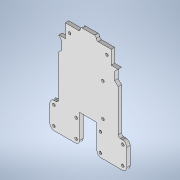
# Autodesk Inventor part: Основа робота
Saved by Autodesk Inventor 2020 (Build 240168000, 168)
## iProperties
Created: 2021-02-28
Part Number: Основа робота
Material: Типовые
Document SubType Name: Обычные детали
Designer: Антон
Density: 1 g/cm^3
Appearance: По умолчанию
Mass: 52.0111 g
Surface Area: 352.197 cm^2
Volume: 52.0111 cm^3
Sheet Metal Rule: По умолчанию
Author: Антон
Autodesk Inventor part; units mm, degrees
ref_plane "YZ Plane" through (0, 0, 0) normal (1, 0, 0) x (0, 1, 0)
ref_plane "XZ Plane" through (0, 0, 0) normal (0, 1, 0) x (-1, 0, 0)
ref_plane "XY Plane" through (0, 0, 0) normal (0, 0, 1) x (1, 0, 0)
sketch "Эскиз1" plane through (0, 0, 0) normal (0, 0, 1) x (1, 0, 0)
  line L0 (0, 0) -> (34.5, 0)
  line L1 (34.5, 0) -> (34.5, 114.55)
  line L2 (34.5, 114.55) -> (0, 114.55)
  line L3 (0, 114.55) -> (0, 0)
  line L4 (0, 0) -> (-9.9, 0)
  line L5 (-9.9, 0) -> (-9.9, 30.3)
  line L6 (-9.9, 30.3) -> (0, 30.3)
  line L7 (0, 30.3) -> (0, 0)
  line L8 (-9.9, 0) -> (-5.35, 0)
  line L9 (-5.35, 0) -> (-5.35, 4.55)
  line L10 (-5.35, 4.55) -> (-5.35, 25.75)
  circle A0 centre (-5.35, 25.75) radius 1.6
  circle A1 centre (-5.35, 4.55) radius 1.6
  line L11 (34.5, 0) -> (24.5, 0)
  line L12 (24.5, 0) -> (24.5, 33)
  line L13 (24.5, 33) -> (34.5, 33)
  line L14 (34.5, 33) -> (34.5, 0)
  line L15 (24.5, 4.55) -> (20.5, 4.55)
  line L16 (24.5, 25.75) -> (20.5, 25.75)
  circle A2 centre (20.5, 25.75) radius 1.6
  circle A3 centre (20.5, 4.55) radius 1.6
  line L17 (34.5, 114.55) -> (34.5, 114.55)
  line L18 (34.5, 114.55) -> (18, 114.55)
  line L19 (20.5, 25.75) -> (20.5, 4.55)
  circle A4 centre (12.95, 106.55) radius 1.6
  line L20 (8, 114.55) -> (8, 98.55)
  line L21 (8, 98.55) -> (0, 98.55)
  line L22 (0, 98.55) -> (0, 129.6)
  line L23 (34.5, 114.55) -> (25.25, 114.55)
  line L24 (25.25, 114.55) -> (25.25, 119)
  line L25 (25.25, 119) -> (34.5, 119)
  line L26 (34.5, 119) -> (34.5, 114.55)
  line L27 (0, 98.55) -> (4, 94.55)
  line L28 (4, 94.55) -> (4, 85.125)
  line L29 (4, 85.125) -> (0, 81.125)
  point P0 (0, 30.3)
  point P1 (34.5, 33)
  point P2 (0, 182.1)
  point P3 (20.5, 15.15)
  point P4 (-5.35, 15.15)
  point P5 (0, 98.55)
  point P6 (8, 106.55)
  point P7 (0, 114.55)
  dimension "d0" = 34.5
  dimension "d1" = 114.55
  dimension "d191" = 9.9
  dimension "d192" = 30.3
  dimension "d207" = 4.55
  dimension "d208" = 4.55
  dimension "d209" = 21.2
  dimension "d210" = 10
  dimension "d211" = 33
  dimension "d215" = 4
  dimension "d290" = 3.2
  dimension "d387" = 21.2
  dimension "d418" = 4.55
  dimension "d421" = 3.2
  dimension "d427" = 8
  dimension "d428" = 16
  dimension "d433" = 4.95
  dimension "d448" = 9.25
  dimension "d450" = 4.45
  dimension "d453" = 45
  dimension "d454" = 4
  dimension "d455" = 17.425
  constraints: 60 end point, 10 parallel, 8 perpendicular, 8 point on line, 6 horizontal, 5 centre point, 4 coincident, 3 equal radius, 3 midpoint, 2 collinear, 2 horizontal alignment, 2 vertical
  measures "d0" distance of L2.end L1.end
  measures "d1" distance of L1.end L0.end
  measures "d191" distance of L5.end L6.end
  measures "d192" distance of L4.end L5.end
  measures "d207" distance of L4.end L8.end
  measures "d208" distance of L8.end L9.end
  measures "d209" distance of L9.end L10.end
  measures "d210" distance of L12.end L13.end
  measures "d211" distance of L11.end L12.end
  measures "d215" distance of L16.start L16.end
  measures "d290" diameter of A2
  measures "d387" distance of L19.end L19.start
  measures "d418" distance from line of L0 L15.end
  measures "d421" diameter of A4
  measures "d427" distance of L20.end L21.end
  measures "d428" distance of L20.start L20.end
  measures "d433" distance of A4.centre point (8, 106.55)
  measures "d448" distance of L24.end L25.end
  measures "d450" distance of L23.end L24.end
  measures "d453" angle of L3 L29
  measures "d454" distance between parallel lines of L3 L28
  measures "d455" distance of L21.end L29.end
extrude "Выдавливание1" add sketch "Эскиз1" along normal blind 4 contours L3 L29 L28 L27 L21 L20 L2 L1 L13 L12 L16 A2 L19 A3 L15 L0 | L4 L5 L6 L3 | L15 A3 L19 A2 L16 L12 | L2 L24 L25 L26
mirror "Зеркальное отражение1" about plane through (34.5, 33, 0) normal (1, 0, 0)
sketch "Эскиз32" plane through (0, 0, 4) normal (0, 0, 1) x (1, 0, 0)
  line L0 (24.5, 33) -> (34.5, 33) construction
  line L1 (34.5, 33) -> (34.5, 39.862) construction
  line L2 (34.5, 39.862) -> (51.4, 39.862) construction
  line L3 (51.4, 39.862) -> (51.4, 78.087) construction
  point P0 (0, 0)
  point P1 (44.5, 33)
  dimension "d434" = 6.862
  dimension "d435" = 16.9
  dimension "d451" = 38.225
  constraints: 7 end point, 2 vertical, 1 horizontal
  measures "d434" distance of L0.end L1.end
  measures "d435" distance of L1.end L2.end
  measures "d451" distance of L2.end L3.end
hole "Отверстие14" at (51.4, 39.862, 4) at (51.4, 78.087, 4) direction (0, 0, -1) diameter 3.2 end through all
fillet "Сопряжение13" radius 2.225 4 edges at (25.25, 114.55, 2) (25.25, 119, 2) (43.75, 114.55, 2) (43.75, 119, 2)
fillet "Сопряжение2" radius 5.05 6 edges at (-9.9, 30.3, 2) (-9.9, 0, 2) (24.5, 0, 2) (44.5, 0, 2) (78.9, 0, 2) (78.9, 30.3, 2)
sketch "Эскиз19" plane through (0, 0, 0) normal (0, 0, -1) x (-1, 0, 0)
  line L0 (-15.75, 108.1666) -> (-12.95, 109.7832)
  line L1 (-12.95, 109.7832) -> (-10.15, 108.1666)
  line L2 (-10.15, 108.1666) -> (-10.15, 104.9334)
  line L3 (-10.15, 104.9334) -> (-12.95, 103.3168)
  line L4 (-12.95, 103.3168) -> (-15.75, 104.9334)
  line L5 (-15.75, 104.9334) -> (-15.75, 108.1666)
  line L6 (0, 81.125) -> (0, 30.3) projected
  circle A0 centre (-12.95, 106.55) radius 1.6 projected
  point P0 (0, 139.6)
  point P1 (-78, 139.6)
  point P2 (-14, 129.6)
  point P3 (-64, 129.6)
  point P4 (0, 119.25)
  point P5 (0, 97.45)
  point P6 (0, 129.6)
  point P7 (-78, 129.6)
  point P8 (-8, 114.55)
  point P9 (-61, 114.55)
  dimension "d423" = 5.6
  constraints: 12 end point, 1 coincident, 1 parallel, 14 other
  measures "d423" distance between parallel lines of L2 L5
extrude "Выдавливание7" cut sketch "Эскиз19" against normal blind 2.6 contours L0 L1 L2 L3 L4 L5 | A0
fillet "Сопряжение12" radius 2.725 2 edges at (69, 30.3, 2) (0, 30.3, 2)
sketch "Эскиз25" plane through (0, 0, 0) normal (0, 0, -1) x (-1, 0, 0)
  circle A0 centre (-20.5, 25.75) radius 1.6 projected
  circle A1 centre (-20.5, 4.55) radius 1.6 projected
  circle A2 centre (5.35, 25.75) radius 1.6 projected
  circle A3 centre (5.35, 4.55) radius 1.6 projected
  circle A4 centre (-48.5, 25.75) radius 1.6 projected
  circle A5 centre (-48.5, 4.55) radius 1.6 projected
  circle A6 centre (-74.35, 4.55) radius 1.6 projected
  circle A7 centre (-74.35, 25.75) radius 1.6 projected
  circle A8 centre (-56.05, 106.55) radius 1.6 projected
  circle A9 centre (-56.05, 106.55) radius 1.6 projected
  circle A10 centre (-51.4, 39.862) radius 1.6 projected
  circle A11 centre (-51.4, 39.862) radius 1.6 projected
  circle A12 centre (-51.4, 78.087) radius 1.6 projected
  point P0 (0, 0)
  constraints: 11 coincident
pattern_sketch "Массив по эскизу1" of "Выдавливание7" from (12.95, 106.55, 0) copies at (20.5, 25.75, 0) at (20.5, 4.55, 0) at (-5.35, 25.75, 0) at (-5.35, 4.55, 0) at (48.5, 25.75, 0) at (48.5, 4.55, 0) at (74.35, 4.55, 0) at (74.35, 25.75, 0) at (56.05, 106.55, 0) at (51.4, 39.862, 0) at (51.4, 78.087, 0)
fillet "Сопряжение11" radius 0.2 1 edges at (0, 98.55, 2)
sketch "Эскиз31" plane through (0, 0, 0) normal (0, 0, -1) x (-1, 0, 0)
  line L0 (-69, 98.55) -> (0, 98.55) construction
  line L1 (0, 98.55) -> (0, 33) construction
  line L2 (0, 33) -> (-69, 33) construction
  line L3 (-69, 33) -> (-69, 98.55) construction
  line L4 (-61, 98.55) -> (-69, 98.55) projected
  line L5 (-69, 81.125) -> (-69, 30.3) projected
  line L6 (0, 81.125) -> (0, 30.3) projected
  line L7 (-24.5, 33) -> (-44.5, 33) projected
  point P0 (0, 0)
  point P1 (-69, 97.45)
  point P2 (-69, 32.99)
  point P3 (0, 97.45)
  point P4 (-34.5, 33)
  constraints: 3 collinear, 1 horizontal, 3 other
equation "\"Радиус_гибки\" = Толщина"
equation "\"Ширина_просечки\" = Толщина"
equation "\"Глубина_просечки\" = 0.5 * Толщина"
equation "\"Размер_просечки\" = 4 * Толщина"
equation "\"Мин_остаток\" = 2 * Толщина"
equation "\"Радиус_перехода\" = Радиус_гибки"
equation "\"Радиус_Якоби\" = Толщина"
equation "\"Размер_зазора\" = Толщина"
equation "\"Гайка_М3_з\" = 5.6"
equation "\"d130\" = 5.6"
equation "\"Толщина\" = 0.5"
